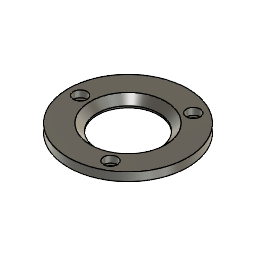
OpenATC-Body-top-cover-development (Autodesk Fusion 360 design; units mm, degrees)
Autodesk Fusion 360 part; units mm, degrees
sketch "Sketch1" plane through (0, 0, 0) normal (0, 0, 1) x (1, 0, 0)
  circle A0 centre (0, 0) radius 18
  circle A1 centre (0, 0) radius 35
  dimension "d1" = 36
  dimension "d2" = 70
  constraint coincident A0.centre A1.centre
  measures "d1" diameter of A0
  measures "d2" diameter of A1
extrude "Extrude1" add sketch "Sketch1" along normal blind 5
sketch "Sketch2" plane through (0, 0, 5) normal (0, 0, 1) x (-1, 0, 0)
  circle A0 centre (0, 0) radius 18
  circle A1 centre (0, 0) radius 35
  line L0 (0, 0) -> (28, 0) construction
  line L1 (0, 0) -> (-14, -24.2487) construction
  line L2 (0, 0) -> (-14, 24.2487) construction
  dimension "d5" = 28
  dimension "d8" = 28
  dimension "d13" = 120
  dimension "d14" = 28
  dimension "d15" = 120
  constraint coincident A0.centre A1.centre
  constraint horizontal L0
  measures "d5" distance of A0.centre L0.end
  measures "d8" distance of A0.centre L1.end
  measures "d13" angle of L0 L1
  measures "d14" distance of A0.centre L2.end
  measures "d15" angle of L1 L2
hole "Hole1" at (-28, 0, 5) at (14, -24.2487, 5) at (14, 24.2487, 5) direction (0, 0, -1) diameter 4.5 end through all counterbore diameter 8 counterbore depth 4
chamfer "Chamfer1" distance 4 angle 45 1 edges at (-16.7819, 6.5091, 5)
equation "d8 = d5"
equation "d14 = d5"
equation "d15 = d13"
